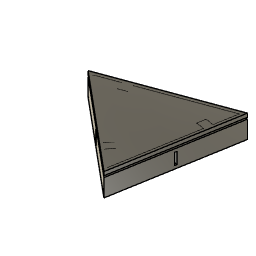
TreeNode v1 aka 1.2 (Autodesk Fusion 360 design; units mm, degrees)
Autodesk Fusion 360 part; units mm, degrees
sketch "base" plane through (0, 0, 0) normal (0, 0, 1) x (1, 0, 0)
  line L0 (0, 0) -> (107.551, -89.6258)
  line L1 (107.551, -89.6258) -> (131.3937, 48.329)
  line L2 (131.3937, 48.329) -> (0, 0)
  line L3 (-7.0948, 1.2262) -> (110.0365, -96.3832)
  line L4 (110.0365, -96.3832) -> (136.0031, 53.8602)
  line L5 (136.0031, 53.8602) -> (-7.0948, 1.2262)
  dimension "d1" = 140
  dimension "d2" = 3.6
  dimension "d3" = 3.6
  dimension "d4" = 3.6
  constraint coincident L0.start L2.end
  constraint parallel L0 L3
  constraint parallel L2 L5
  constraint parallel L1 L4
  measures "d1" distance of L0.start L0.end
  measures "d2" distance of L0 L3
  measures "d3" distance of L1 L4
  measures "d4" distance of L2 L5
extrude "Extrude4" add sketch "base" against normal blind 1.6 contours L0 L1 L2 | L3 L4 L5 makes body 1
extrude "Extrude5" add sketch "base" along normal blind 20 bodies 1
sketch "edge1" plane through (119.4724, -20.6484, 0) normal (-0.985391, 0.170305, 0) x (-0.170305, -0.985391, 0)
  line L0 (-70, 0) -> (70, 0)
  line L1 (70, 0) -> (70, 20)
  line L2 (70, 20) -> (-70, 20)
  line L3 (-70, 20) -> (-70, 0)
  line L4 (-58, 13) -> (-52, 13)
  line L5 (-52, 13) -> (-52, 7)
  line L6 (-52, 7) -> (-58, 7)
  line L7 (-58, 7) -> (-58, 13)
  line L8 (-58, 13) -> (-52, 7) construction
  line L9 (-52, 13) -> (-58, 7) construction
  line L10 (0, 20) -> (0, 0)
  line L11 (58, 13) -> (52, 13)
  line L12 (58, 7) -> (58, 13)
  line L13 (52, 7) -> (58, 7)
  line L14 (52, 13) -> (52, 7)
  point P0 (-67.5, 10)
  point P1 (-70, 10)
  point P2 (-57.5, 10)
  point P3 (-45, 10)
  point P4 (-60, 10)
  point P5 (-62.5, 10)
  point P6 (-65, 10)
  point P7 (-55, 10)
  point P8 (-52.5, 10)
  point P9 (-50, 10)
  point P10 (-47.5, 10)
  point P11 (-55, 10)
  point P12 (0, 20)
  point P13 (55, 10)
  point P14 (57.5, 10)
  point P15 (52.5, 10)
  point P16 (70, 10)
  point P17 (50, 10)
  point P18 (47.5, 10)
  point P19 (45, 10)
  point P20 (60, 10)
  point P21 (62.5, 10)
  point P22 (65, 10)
  point P23 (67.5, 10)
  dimension "d18" = 6
  dimension "d19" = 6
  constraint midpoint L3 P1
  constraint horizontal L4
  constraint perpendicular L4 L5
  constraint parallel L4 L6
  constraint parallel L5 L7
  constraint coincident L8 P11
  constraint coincident L9 P11
  constraint coincident P11 P7
  constraint midpoint L2 P12
  constraint coincident L10.end origin
  constraint coincident P12 L10.start
  constraint symmetric P0 L10 P23
  constraint symmetric P1 L10 P16
  constraint symmetric P2 L10 P14
  constraint symmetric P3 L10 P19
  constraint symmetric P4 L10 P20
  constraint symmetric P5 L10 P21
  constraint symmetric P6 L10 P22
  constraint symmetric P8 L10 P15
  constraint symmetric P9 L10 P17
  constraint symmetric P10 L10 P18
  constraint symmetric L4.start L10 L11.start
  constraint symmetric L4.end L10 L11.end
  constraint symmetric L5.end L10 L13.start
  constraint symmetric L6.end L10 L12.start
  constraint symmetric P11 L10 P13
  measures "d18" distance of L5.end L6.end
  measures "d19" distance of L4.end L5.end
extrude "Extrude9" cut sketch "edge1" against normal blind 2.1 contours L4 L5 L6 L7 bodies 1
extrude "Extrude10" cut sketch "edge1" against normal blind 2.1 contours L11 L12 L13 L14 bodies 1
sketch "edge2" plane through (0, 0, 0) normal (0.345207, -0.938527, 0) x (0.938527, 0.345207, 0)
  line L0 (0, 0) -> (140, 0)
  line L1 (140, 0) -> (140, 20)
  line L2 (140, 20) -> (0, 20)
  line L3 (0, 20) -> (0, 0)
  line L4 (0, 10) -> (69, 10)
  line L5 (69, 10) -> (128, 10)
  line L6 (128, 10) -> (140, 10)
  line L7 (122, 13) -> (128, 13)
  line L8 (128, 13) -> (128, 7)
  line L9 (128, 7) -> (122, 7)
  line L10 (122, 7) -> (122, 13)
  line L11 (122, 13) -> (128, 7) construction
  line L12 (128, 13) -> (122, 7) construction
  line L13 (12, 13) -> (18, 13)
  line L14 (18, 13) -> (18, 7)
  line L15 (18, 7) -> (12, 7)
  line L16 (12, 7) -> (12, 13)
  line L17 (12, 13) -> (18, 7) construction
  line L18 (18, 13) -> (12, 7) construction
  point P0 (0, 10)
  point P1 (15, 10)
  point P2 (140, 10)
  point P3 (125, 10)
  point P4 (140, 10)
  point P5 (125, 10)
  point P6 (15, 10)
  dimension "d34" = 15
  dimension "d35" = 15
  dimension "d36" = 6
  dimension "d37" = 6
  dimension "d38" = 6
  dimension "d39" = 6
  constraint midpoint L3 P0
  constraint perpendicular L3 L4
  constraint perpendicular L1 L5
  constraint midpoint L1 P4
  constraint coincident P0 L4.start
  constraint coincident L4 P6
  constraint coincident P4 P2
  constraint coincident L5 P5
  constraint horizontal L7
  constraint perpendicular L7 L8
  constraint parallel L7 L9
  constraint parallel L8 L10
  constraint coincident L11 P5
  constraint coincident L12 P5
  constraint coincident P5 P3
  constraint horizontal L13
  constraint perpendicular L13 L14
  constraint parallel L13 L15
  constraint parallel L14 L16
  constraint coincident L17 P6
  constraint coincident L18 P6
  constraint coincident P6 P1
  measures "d34" distance of P0 P6
  measures "d35" distance of P5 P4
  measures "d36" distance of L8.end L9.end
  measures "d37" distance of L7.end L8.end
  measures "d38" distance of L14.end L15.end
  measures "d39" distance of L13.end L14.end
sketch "edge3" plane through (0, 0, 0) normal (0.640184, 0.768221, 0) x (-0.768221, 0.640184, 0)
  line L0 (-140, 0) -> (0, 0)
  line L1 (0, 0) -> (0, 20)
  line L2 (0, 20) -> (-140, 20)
  line L3 (-140, 20) -> (-140, 0)
  line L4 (-140, 10) -> (-80, 10)
  line L5 (-80, 10) -> (0, 10)
  line L6 (-18, 13) -> (-12, 13)
  line L7 (-12, 13) -> (-12, 7)
  line L8 (-12, 7) -> (-18, 7)
  line L9 (-18, 7) -> (-18, 13)
  line L10 (-18, 13) -> (-12, 7) construction
  line L11 (-12, 13) -> (-18, 7) construction
  line L12 (-122, 7) -> (-128, 7)
  line L13 (-128, 7) -> (-128, 13)
  line L14 (-128, 13) -> (-122, 13)
  line L15 (-122, 13) -> (-122, 7)
  line L16 (-122, 7) -> (-128, 13) construction
  line L17 (-128, 7) -> (-122, 13) construction
  point P0 (0, 10)
  point P1 (-15, 10)
  point P2 (-140, 10)
  point P3 (-125, 10)
  point P4 (-140, 10)
  point P5 (-15, 10)
  point P6 (-125, 10)
  dimension "d40" = 15
  dimension "d41" = 15
  dimension "d42" = 6
  dimension "d43" = 6
  dimension "d44" = 6
  dimension "d45" = 6
  constraint midpoint L3 P4
  constraint perpendicular L3 L4
  constraint midpoint L1 P0
  constraint perpendicular L1 L5
  constraint coincident P0 L5.end
  constraint coincident L5 P5
  constraint coincident P4 P2
  constraint coincident L4 P6
  constraint horizontal L6
  constraint perpendicular L6 L7
  constraint parallel L6 L8
  constraint parallel L7 L9
  constraint coincident L10 P5
  constraint coincident L11 P5
  constraint coincident P5 P1
  constraint horizontal L12
  constraint perpendicular L12 L13
  constraint parallel L12 L14
  constraint parallel L13 L15
  constraint coincident L16 P6
  constraint coincident L17 P6
  constraint coincident P6 P3
  measures "d40" distance of P6 P4
  measures "d41" distance of P0 P5
  measures "d42" distance of L7.end L8.end
  measures "d43" distance of L6.end L7.end
  measures "d44" distance of L13.end L14.end
  measures "d45" distance of L12.end L13.end
extrude "Extrude11" cut sketch "edge3" against normal blind 2.1 contours L4 L13 L14 L15 | L4 L12 L13 L15 bodies 1
extrude "Extrude12" cut sketch "edge3" against normal blind 2.1 contours L5 L7 L8 L9 | L5 L6 L7 L9 bodies 1
extrude "Extrude13" cut sketch "edge2" against normal blind 2.1 contours L4 L13 L14 L16 | L4 L14 L15 L16 bodies 1
extrude "Extrude14" cut sketch "edge2" against normal blind 2.1 contours L5 L8 L9 L10 | L5 L7 L8 L10 bodies 1
sketch "outEdge1" plane through (-2.3047, -2.7656, 0) normal (-0.640184, -0.768221, 0) x (0.768221, -0.640184, 0)
  line L0 (-6.2354, 20) -> (-6.2354, -1.6)
  line L1 (-6.2354, -1.6) -> (146.2354, -1.6)
  line L2 (146.2354, -1.6) -> (146.2354, 20)
  line L3 (146.2354, 20) -> (-6.2354, 20)
  line L4 (-6.2354, 9.2) -> (146.2354, 9.2)
  line L5 (70, 20) -> (70, -1.6)
  line L6 (71.5, 16.3) -> (68.5, 16.3)
  line L7 (68.5, 16.3) -> (68.5, 2.1)
  line L8 (68.5, 2.1) -> (71.5, 2.1)
  line L9 (71.5, 2.1) -> (71.5, 16.3)
  line L10 (71.5, 16.3) -> (68.5, 2.1) construction
  line L11 (68.5, 16.3) -> (71.5, 2.1) construction
  point P0 (70, 9.2)
  point P1 (70, 9.2)
  dimension "d54" = 3
  dimension "d55" = 14.2
  constraint midpoint L0 L4.start
  constraint midpoint L2 L4.end
  constraint midpoint L3 L5.start
  constraint midpoint L1 L5.end
  constraint midpoint L5 P1
  constraint horizontal L6
  constraint perpendicular L6 L7
  constraint parallel L6 L8
  constraint parallel L7 L9
  constraint coincident L10 P1
  constraint coincident L11 P1
  constraint coincident P1 P0
  measures "d54" distance of L7.end L8.end
  measures "d55" distance of L6.end L7.end
extrude "Extrude15" cut sketch "outEdge1" against normal blind 3.6 contours L4 L5 L6 L7 | L4 L5 L7 L8 | L4 L5 L6 L9 | L4 L5 L8 L9 bodies 1
sketch "outEdge2" plane through (123.0198, -21.2615, 0) normal (0.985391, -0.170305, 0) x (0.170305, 0.985391, 0)
  line L0 (-76.2354, 20) -> (-76.2354, -1.6)
  line L1 (-76.2354, -1.6) -> (76.2354, -1.6)
  line L2 (76.2354, -1.6) -> (76.2354, 20)
  line L3 (76.2354, 20) -> (-76.2354, 20)
  line L4 (-76.2354, 9.2) -> (76.2354, 9.2)
  line L5 (0, 20) -> (0, -1.6)
  line L6 (1.5, 2.1) -> (-1.5, 2.1)
  line L7 (-1.5, 2.1) -> (-1.5, 16.3)
  line L8 (-1.5, 16.3) -> (1.5, 16.3)
  line L9 (1.5, 16.3) -> (1.5, 2.1)
  line L10 (1.5, 2.1) -> (-1.5, 16.3) construction
  line L11 (-1.5, 2.1) -> (1.5, 16.3) construction
  point P0 (0, 9.2)
  point P1 (0, 9.2)
  dimension "d58" = 3
  dimension "d59" = 14.2
  constraint midpoint L0 L4.start
  constraint midpoint L2 L4.end
  constraint midpoint L3 L5.start
  constraint midpoint L1 L5.end
  constraint midpoint L4 P1
  constraint horizontal L6
  constraint perpendicular L6 L7
  constraint parallel L6 L8
  constraint parallel L7 L9
  constraint coincident L10 P1
  constraint coincident L11 P1
  constraint coincident P1 P0
  measures "d58" distance of L7.end L8.end
  measures "d59" distance of L6.end L7.end
sketch "outEdge3" plane through (-1.2427, 3.3787, 0) normal (-0.345207, 0.938527, 0) x (-0.938527, -0.345207, 0)
  line L0 (-146.2354, 20) -> (-146.2354, -1.6)
  line L1 (-146.2354, -1.6) -> (6.2354, -1.6)
  line L2 (6.2354, -1.6) -> (6.2354, 20)
  line L3 (6.2354, 20) -> (-146.2354, 20)
  line L4 (-146.2354, 9.2) -> (6.2354, 9.2)
  line L5 (-70, 20) -> (-70, -1.6)
  line L6 (-68.5, 2.1) -> (-71.5, 2.1)
  line L7 (-71.5, 2.1) -> (-71.5, 16.3)
  line L8 (-71.5, 16.3) -> (-68.5, 16.3)
  line L9 (-68.5, 16.3) -> (-68.5, 2.1)
  line L10 (-68.5, 2.1) -> (-71.5, 16.3) construction
  line L11 (-71.5, 2.1) -> (-68.5, 16.3) construction
  point P0 (-70, 9.2)
  point P1 (-70, 9.2)
  dimension "d60" = 3
  dimension "d61" = 14.2
  constraint midpoint L0 L4.start
  constraint midpoint L2 L4.end
  constraint midpoint L3 L5.start
  constraint midpoint L1 L5.end
  constraint midpoint L5 P1
  constraint horizontal L6
  constraint perpendicular L6 L7
  constraint parallel L6 L8
  constraint parallel L7 L9
  constraint coincident L10 P1
  constraint coincident L11 P1
  constraint coincident P1 P0
  measures "d60" distance of L7.end L8.end
  measures "d61" distance of L6.end L7.end
extrude "Extrude16" cut sketch "outEdge2" against normal blind 3.6 contours L4 L5 L7 L8 | L4 L5 L6 L7 | L4 L5 L8 L9 | L4 L5 L6 L9 bodies 1
extrude "Extrude17" cut sketch "outEdge3" against normal blind 3.6 contours L4 L5 L7 L8 | L4 L5 L6 L7 | L4 L5 L8 L9 | L4 L5 L6 L9 bodies 1
sketch "capFixator" plane through (0, 0, 20) normal (0, 0, 1) x (-1, 0, 0)
  line L0 (0, 0) -> (-131.3937, -48.329)
  line L1 (-131.3937, -48.329) -> (-107.551, 89.6258)
  line L2 (-107.551, 89.6258) -> (0, 0)
  line L3 (-136.0031, -53.8602) -> (7.0948, -1.2262)
  line L4 (7.0948, -1.2262) -> (-110.0365, 96.3832)
  line L5 (-110.0365, 96.3832) -> (-136.0031, -53.8602)
  line L6 (-86.0408, 71.7007) -> (-92.4426, 64.0184)
  line L7 (-82.9679, 69.1399) -> (-86.0408, 71.7007)
  line L8 (-26.2787, -9.6658) -> (-29.7308, -0.2805)
  line L9 (-30.0329, -11.0466) -> (-26.2787, -9.6658)
  line L10 (-86.0408, 71.7007) -> (-92.4426, 64.0184)
  line L11 (-92.4426, 64.0184) -> (-84.7604, 57.6166)
  line L12 (-84.7604, 57.6166) -> (-78.3586, 65.2988)
  line L13 (-78.3586, 65.2988) -> (-86.0408, 71.7007)
  line L14 (-26.2787, -9.6658) -> (-35.664, -13.1179)
  line L15 (-35.664, -13.1179) -> (-39.1161, -3.7326)
  line L16 (-39.1161, -3.7326) -> (-29.7308, -0.2805)
  line L17 (-29.7308, -0.2805) -> (-26.2787, -9.6658)
  line L18 (-126.6252, -20.738) -> (-124.9221, -10.8841)
  line L19 (-124.9221, -10.8841) -> (-115.0682, -12.5872)
  line L20 (-115.0682, -12.5872) -> (-116.7713, -22.4411)
  line L21 (-116.7713, -22.4411) -> (-126.6252, -20.738)
  point P0 (-107.551, 89.6258)
  point P1 (-14.4509, -5.3153)
  point P2 (-82.1997, 68.4997)
  point P3 (-86.0408, 71.7007)
  point P4 (-78.3586, 65.2988)
  point P5 (-92.4426, 64.0184)
  point P6 (-30.9714, -11.3918)
  point P7 (-26.2787, -9.6658)
  point P8 (-35.664, -13.1179)
  point P9 (-29.7308, -0.2805)
  point P10 (-125.7736, -15.8111)
  point P11 (-131.3937, -48.329)
  point P12 (-126.6252, -20.738)
  point P13 (-124.9221, -10.8841)
  point P14 (-116.7713, -22.4411)
  dimension "d67" = 15.3974
  dimension "d75" = 33
  dimension "d76" = 5
  dimension "d77" = 5
  dimension "d78" = 10
  dimension "d79" = 33
  dimension "d80" = 5
  dimension "d81" = 5
  dimension "d82" = 10
  dimension "d121" = 33
  dimension "d122" = 5
  dimension "d123" = 5
  dimension "d124" = 10
  constraint coincident P0 L1.end
  constraint coincident L0.start L2.end
  constraint coincident L0 P1
  constraint coincident L2 P2
  constraint coincident L2 P3
  constraint coincident L2 P4
  constraint coincident P3 L6.start
  constraint coincident P5 L6.end
  constraint coincident L0 P6
  constraint coincident L0 P7
  constraint coincident L0 P8
  constraint coincident P7 L8.start
  constraint coincident P9 L8.end
  constraint perpendicular L10 L11
  constraint parallel L10 L12
  constraint parallel L11 L13
  constraint perpendicular L7 L10
  constraint perpendicular L14 L15
  constraint parallel L14 L16
  constraint parallel L15 L17
  constraint coincident P8 L14.end
  constraint coincident L1 P10
  constraint coincident L1 P12
  constraint coincident L1 P13
  constraint coincident P12 L18.start
  constraint perpendicular L18 L19
  constraint parallel L18 L20
  constraint parallel L19 L21
  constraint coincident P13 L18.end
  measures "d67" distance of L0.start P1
  measures "d75" distance of P0 P2
  measures "d76" distance of P2 P3
  measures "d77" distance of P2 P4
  measures "d78" distance of P3 P5
  measures "d79" distance of L0.start P6
  measures "d80" distance of P6 P7
  measures "d81" distance of P6 P8
  measures "d82" distance of P7 P9
  measures "d121" distance of P10 P11
  measures "d122" distance of P10 P12
  measures "d123" distance of P10 P13
  measures "d124" distance of P12 P14
extrude "Extrude18" add sketch "capFixator" against normal blind 3.6 contours L0 L8 L9 L14 L15 L16 L17 bodies 1
extrude "Extrude19" add sketch "capFixator" against normal blind 3.6 contours L2 L6 L7 L10 L11 L12 L13 bodies 1
sketch "capCutForMagnet" plane through (0, 0, 20) normal (0, 0, 1) x (-1, 0, 0)
  line L0 (-29.7308, -0.2805) -> (-26.2787, -9.6658)
  line L1 (-39.1161, -3.7326) -> (-29.7308, -0.2805)
  line L2 (-35.664, -13.1179) -> (-39.1161, -3.7326)
  line L3 (-26.2787, -9.6658) -> (-29.7308, -0.2805)
  line L4 (-28.6736, -8.9484) -> (-30.7448, -3.3173)
  line L5 (-30.7448, -3.3173) -> (-36.376, -5.3885)
  line L6 (-36.376, -5.3885) -> (-34.3048, -11.0197)
  line L7 (-34.3048, -11.0197) -> (-28.6736, -8.9484)
  line L8 (-92.4426, 64.0184) -> (-84.7604, 57.6166)
  line L9 (-86.0408, 71.7007) -> (-92.4426, 64.0184)
  line L10 (-84.7604, 57.6166) -> (-78.3586, 65.2988)
  line L11 (-85.4646, 69.268) -> (-89.3057, 64.6586)
  line L12 (-89.3057, 64.6586) -> (-84.6964, 60.8175)
  line L13 (-84.6964, 60.8175) -> (-80.8553, 65.4268)
  line L14 (-80.8553, 65.4268) -> (-85.4646, 69.268)
  line L15 (-115.0682, -12.5872) -> (-116.7713, -22.4411)
  line L16 (-116.7713, -22.4411) -> (-126.6252, -20.738)
  line L17 (-124.9221, -10.8841) -> (-115.0682, -12.5872)
  line L18 (-124.8065, -19.0227) -> (-118.8941, -20.0445)
  line L19 (-118.8941, -20.0445) -> (-117.8723, -14.1322)
  line L20 (-117.8723, -14.1322) -> (-123.7846, -13.1103)
  line L21 (-123.7846, -13.1103) -> (-124.8065, -19.0227)
  point P0 (-32.5248, -7.1685)
  point P1 (-28.6736, -8.9484)
  point P2 (-36.376, -5.3885)
  point P3 (-30.7448, -3.3173)
  point P4 (-85.0805, 65.0427)
  point P5 (-85.4646, 69.268)
  point P6 (-89.3057, 64.6586)
  point P7 (-84.6964, 60.8175)
  point P8 (-121.3394, -16.5774)
  point P9 (-124.8065, -19.0227)
  point P10 (-118.8941, -20.0445)
  point P11 (-117.8723, -14.1322)
  dimension "d87" = 5
  dimension "d88" = 5.5
  dimension "d89" = 2
  dimension "d90" = 8.5
  dimension "d91" = 2
  dimension "d92" = 2.5
  dimension "d93" = 2.5
  dimension "d94" = 2
  dimension "d97" = 5.5
  dimension "d98" = 5
  dimension "d99" = 2.5
  dimension "d100" = 2.5
  dimension "d101" = 2
  dimension "d102" = 2
  dimension "d103" = 2
  dimension "d104" = 8.5
  dimension "d129" = 5.5
  dimension "d130" = 2.5
  dimension "d131" = 2.5
  dimension "d132" = 5
  dimension "d133" = 2
  dimension "d134" = 2
  dimension "d135" = 8.5
  dimension "d136" = 2
  constraint perpendicular L4 L5
  constraint parallel L4 L6
  constraint parallel L5 L7
  constraint coincident P3 L4.end
  constraint parallel L3 L4
  constraint coincident P1 L4.start
  constraint perpendicular L11 L12
  constraint parallel L11 L13
  constraint parallel L12 L14
  constraint coincident P6 L11.end
  constraint coincident P5 L11.start
  constraint perpendicular L18 L19
  constraint parallel L18 L20
  constraint parallel L19 L21
  constraint coincident P10 L18.end
  constraint coincident P9 L18.start
  measures "d87" distance of P0 L0
  measures "d88" distance of P0 L1
  measures "d89" distance of L0 P1
  measures "d90" distance of L1 P1
  measures "d91" distance of P2 L2
  measures "d92" distance of L1 P2
  measures "d93" distance of L1 P3
  measures "d94" distance of P3 L3
  measures "d97" distance of P4 L8
  measures "d98" distance of P4 L9
  measures "d99" distance of P7 L8
  measures "d100" distance of P6 L8
  measures "d101" distance of P6 L9
  measures "d102" distance of P5 L9
  measures "d103" distance of P7 L10
  measures "d104" distance of P5 L8
  measures "d129" distance of P8 L15
  measures "d130" distance of P11 L15
  measures "d131" distance of P10 L15
  measures "d132" distance of P8 L16
  measures "d133" distance of P10 L16
  measures "d134" distance of P9 L16
  measures "d135" distance of P9 L15
  measures "d136" distance of P11 L17
extrude "Extrude25" cut sketch "capCutForMagnet" against normal blind 2.2 contours L4 L5 L6 L7 bodies 1
extrude "Extrude26" cut sketch "capCutForMagnet" against normal blind 2.2 contours L11 L12 L13 L14 bodies 1
fillet "Fillet1" radius 7 1 edges at (82.1997, -68.4997, 16.4) on bodies 1
fillet "Fillet2" radius 7 1 edges at (30.9714, 11.3918, 16.4) on bodies 1
extrude "Extrude27" add sketch "capFixator" against normal blind 3.7 contours L1 L18 L19 L20 L21 bodies 1
fillet "Fillet3" radius 7 1 edges at (125.7736, 15.8111, 16.3) on bodies 1
extrude "Extrude28" cut sketch "capCutForMagnet" against normal blind 2.2 contours L18 L19 L20 L21 bodies 1
extrude "Extrude29" add sketch "base" along normal blind 0.8 separate body contours L0 L1 L2 | L3 L4 L5 makes body 2
extrude "Extrude30" add sketch "base" against normal blind 3.6 bodies 2
move_body "Move3" bodies 2 to x (1, 0, 0) y (0, 1, 0) z (0, 0, 1) at (0, 0, 23.6)
extrude "Extrude41" add sketch "capFixator" along normal blind 3.6 contours L1 L18 L19 L20 L21 bodies 2
extrude "Extrude42" add sketch "capFixator" along normal blind 3.6 contours L0 L8 L9 L14 L15 L16 L17 bodies 2
extrude "Extrude43" add sketch "capFixator" along normal blind 3.6 contours L2 L6 L7 L10 L11 L12 L13 bodies 2
extrude "Extrude44" cut sketch "capCutForMagnet" along normal blind 2.2 bodies 2
move_body "Move4" bodies 2 to x (1, 0, 0) y (0, 1, 0) z (0, 0, 1) at (0, 0, 2)
equation "d18 = ( 3 * 2 ) * 1 mm"
equation "d19 = ( 3 * 2 ) * 1 mm"
equation "d36 = ( 3 * 2 ) * 1 mm"
equation "d37 = ( 3 * 2 ) * 1 mm"
equation "d38 = ( 3 * 2 ) * 1 mm"
equation "d39 = ( 3 * 2 ) * 1 mm"
equation "d42 = ( 3 * 2 ) * 1 mm"
equation "d43 = ( 3 * 2 ) * 1 mm"
equation "d44 = ( 3 * 2 ) * 1 mm"
equation "d45 = ( 3 * 2 ) * 1 mm"
named bodies: "base", "cap"
